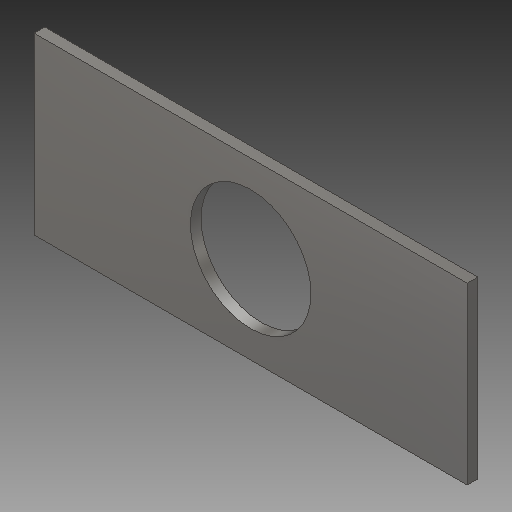
# Autodesk Inventor part: TorquePlate
Saved by Autodesk Inventor 2019.3 (Build 233278000, 278)
## iProperties
Created: 2019-01-26
Part Number: TorquePlate
Material: Steel, Mild
Document SubType Name: Modeling
Designer: mark
Density: 7.85 g/cm^3
Appearance: Semi-Polished
Author: mark
Autodesk Inventor part; units mm, degrees
ref_plane "YZ Plane" through (0, 0, 0) normal (1, 0, 0) x (0, 1, 0)
ref_plane "XZ Plane" through (0, 0, 0) normal (0, 1, 0) x (-1, 0, 0)
ref_plane "XY Plane" through (0, 0, 0) normal (0, 0, 1) x (1, 0, 0)
sketch "Sketch1" plane through (0, 0, 0) normal (0, 0, 1) x (1, 0, 0)
  line L0 (0, 0) -> (125.8, 0)
  line L1 (125.8, 0) -> (125.8, 50.75)
  line L2 (125.8, 50.75) -> (0, 50.75)
  line L3 (0, 50.75) -> (0, 0)
  circle A0 centre (62.9, 25.375) radius 17.5
  dimension "d0" = 125.8
  dimension "d1" = 50.75
  dimension "d4" = 35
  dimension "d5" = 62.9
  dimension "d6" = 25.375
  constraints: 8 end point, 3 perpendicular, 1 centre point, 1 horizontal
  measures "d0" distance of L2.end L1.end
  measures "d1" distance of L1.end L0.end
  measures "d4" diameter of A0
  measures "d5" distance from line of L1 A0.centre
  measures "d6" distance from line of L2 A0.centre
extrude "Extrusion1" add sketch "Sketch1" along normal blind 3.1
body "Solid1"
